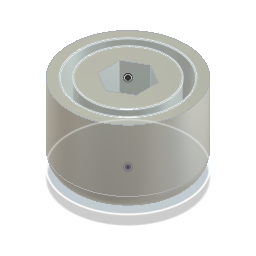
intake+polycarb+holderr (Autodesk Fusion 360 design; units mm, degrees)
Autodesk Fusion 360 part; units mm, degrees
sketch "Sketch1" plane through (0, 0, 0) normal (0, 1, 0) x (1, 0, 0)
  circle A0 centre (0, 0) radius 19.05
  dimension "d1" = 38.1
  constraint coincident A0.centre origin
  measures "d1" diameter of A0
extrude "Extrude1" add sketch "Sketch1" along normal blind 25.4 makes body 1
sketch "Sketch2" plane through (0, 25.4, 0) normal (0, 1, 0) x (-1, 0, 0)
  circle A0 centre (0, 0) radius 19.05
  circle A1 centre (0, 0) radius 12.7
  circle A2 centre (0, 0) radius 15.875
  dimension "d4" = 25.4
  dimension "d5" = 31.75
  constraint coincident A0.centre A1.centre
  measures "d4" diameter of A1
  measures "d5" diameter of A2
extrude "Extrude2" cut sketch "Sketch2" against normal blind 22.225 contours A2 bodies 1
sketch "Sketch3" plane through (0, 0, 0) normal (0, -1, 0) x (1, 0, 0)
  circle A0 centre (0, 0) radius 19.05
  line L0 (6.35, 3.6662) -> (0, 7.3323)
  line L1 (0, 7.3323) -> (-6.35, 3.6662)
  line L2 (-6.35, 3.6662) -> (-6.35, -3.6662)
  line L3 (-6.35, -3.6662) -> (0, -7.3323)
  line L4 (0, -7.3323) -> (6.35, -3.6662)
  line L5 (6.35, -3.6662) -> (6.35, 3.6662)
  line L6 (-11.43, 6.5991) -> (-11.43, -6.5991)
  line L7 (-11.43, -6.5991) -> (0, -13.1982)
  line L8 (0, -13.1982) -> (11.43, -6.5991)
  line L9 (11.43, -6.5991) -> (11.43, 6.5991)
  line L10 (11.43, 6.5991) -> (0, 13.1982)
  line L11 (0, 13.1982) -> (-11.43, 6.5991)
  dimension "d9" = 6.35
  dimension "d17" = 5.08
  constraint coincident A0.centre origin
  measures "d9" distance of A0.centre L5
copy_body "Body->Comp1" bodies 1 removing the originals makes body 2 in component "Component"
extrude "Extrude1'" add sketch "Sketch3" along normal blind 3.175 contours L6 L7 L8 L9 L10 L11 bodies 2 in component "Component"
fillet "Fillet1" radius 5.08 1 edges at (-17.7608, 0, 6.8888) on bodies 2 in component "Component"
fillet "Fillet2" radius 2.54 6 edges at (-5.715, -3.175, 9.8987) (-11.43, -3.175, 0) (-5.715, -3.175, -9.8987) (5.715, -3.175, -9.8987) (5.715, -3.175, 9.8987) (11.43, -3.175, 0) on bodies 2 in component "Component"
sketch "Sketch4" plane through (0, 0, 0) normal (0, 1, 0) x (1, 0, 0)
  line L0 (6.35, 3.6662) -> (0, 7.3323)
  line L1 (0, 7.3323) -> (-6.35, 3.6662)
  line L2 (-6.35, 3.6662) -> (-6.35, -3.6662)
  line L3 (-6.35, -3.6662) -> (0, -7.3323)
  line L4 (0, -7.3323) -> (6.35, -3.6662)
  line L5 (6.35, -3.6662) -> (6.35, 3.6662)
  dimension "d27" = 6.35
  measures "d27" distance of origin L5
extrude "Extrude2'" cut sketch "Sketch4" along normal blind 25.4 bodies 2 in component "Component"
component "Component" placed x (1, 0, 0) y (0, 1, 0) z (0, 0, 1) at (0, 0, 0)
